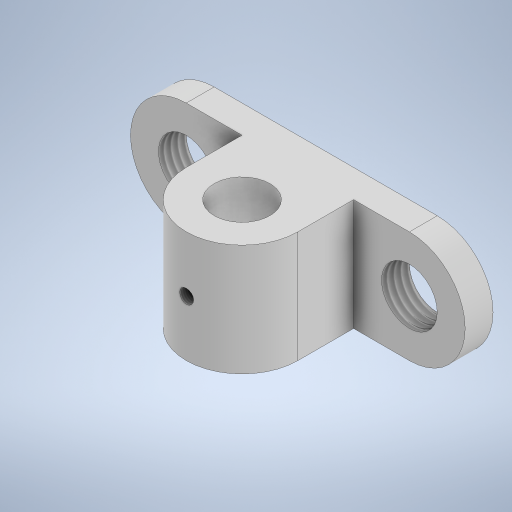
# Autodesk Inventor part: 06022024_ejercicio
Saved by Autodesk Inventor 2024 (Build 280153000, 153)
## iProperties
Created: 2024-02-06
Part Number: 06022024_ejercicio
Material: Generic
Document SubType Name: Modeling
Designer: augus
Density: 1 g/cm^3
Appearance: Default
Author: augus
Autodesk Inventor part; units mm, degrees
ref_plane "YZ Plane" through (0, 0, 0) normal (1, 0, 0) x (0, 1, 0)
ref_plane "XZ Plane" through (0, 0, 0) normal (0, 1, 0) x (-1, 0, 0)
sketch "Sketch2" plane through (0, 0, 0) normal (0, 0, 1) x (1, 0, 0)
  line L0 (-20, 20) -> (20, 20)
  line L1 (20, 20) -> (20, -20)
  line L2 (20, -20) -> (-20, -20)
  line L3 (-20, -20) -> (-20, 20)
  line L4 (-20, 20) -> (20, -20) construction
  line L5 (20, 20) -> (-20, -20) construction
  point P0 (0, 0)
  dimension "d5" = 40
  dimension "d6" = 40
  constraints: 12 end point, 2 midpoint, 2 parallel, 1 horizontal, 1 perpendicular
  measures "d5" distance of L1.end L2.end
  measures "d6" distance of L0.end L1.end
extrude "Extrusion2" add sketch "Sketch2" along normal blind 50
sketch "Sketch3" plane through (20, -20, 0) normal (1, 0, 0) x (0, 0, -1)
  line L0 (0, 40) -> (-50, 40) projected
  line L1 (0, 0) -> (-50, 0) projected
  line L2 (0, 40) -> (-10, 40)
  line L3 (-10, 40) -> (-10, 0)
  line L4 (-10, 0) -> (0, 0)
  line L5 (0, 0) -> (0, 40)
  point P0 (0, 20)
  dimension "d9" = 10
  constraints: 8 end point, 2 parallel, 1 horizontal, 1 perpendicular, 1 point on line
  measures "d9" distance of L4.end L3.end
extrude "Extrusion3" add sketch "Sketch3" along normal blind 40
sketch "Sketch4" plane through (-20, -20, 0) normal (-1, 0, 0) x (0, 0, 1)
  line L0 (0, 40) -> (0, 0) projected
  line L1 (0, 40) -> (50, 40) projected
  line L2 (0, 0) -> (10, 0)
  line L3 (10, 0) -> (10, 40)
  line L4 (10, 40) -> (0, 40)
  line L5 (0, 40) -> (0, 0)
  point P0 (0, 20)
  dimension "d13" = 10
  constraints: 8 end point, 2 parallel, 1 horizontal, 1 perpendicular, 1 point on line
  measures "d13" distance of L4.end L3.end
extrude "Extrusion4" add sketch "Sketch4" along normal blind 40
sketch "Sketch5" plane through (-20, -20, 10) normal (0, 0, 1) x (1, 0, 0)
  line L0 (0, 40) -> (0, 0) projected
  line L1 (-40, 0) -> (80, 0) projected
  line L2 (-20, 40) -> (-40, 40)
  line L3 (-40, 40) -> (-40, 0)
  line L4 (-40, 0) -> (-20, 0)
  line L5 (0, 0) -> (0, 40)
  circle A0 centre (-20, 20) radius 10
  arc A1 (-20, 40) -> (-20, 0) centre (-20, 20) ccw
  line L6 (0, 40) -> (-40, 40) projected
  line L7 (0, 0) -> (-40, 0) projected
  line L8 (-40, 0) -> (-40, 40) projected
  line L9 (60, 0) -> (80, 0)
  line L10 (80, 0) -> (80, 40)
  line L11 (80, 40) -> (60, 40)
  circle A2 centre (60, 20) radius 10
  arc A3 (60, 0) -> (60, 40) centre (60, 20) ccw
  line L12 (40, 40) -> (80, 40) projected
  line L13 (80, 40) -> (80, 0) projected
  line L14 (40, 0) -> (80, 0) projected
  point P0 (20, 20)
  point P1 (80, 20)
  point P2 (-40, 20)
  constraints: 14 end point, 6 tangent, 5 perpendicular, 4 centre point, 4 point on circle, 3 parallel, 2 coincident, 1 horizontal
extrude "Extrusion5" cut sketch "Sketch5" against normal through all contours A3 L11 L10 | A3 L10 L1 | A1 L3 L2 | L1 L3 A1 | A0 | A2
sketch "Sketch6" plane through (-20, -20, 50) normal (0, -1, 0) x (1, 0, 0)
  line L0 (0, -40) -> (-20, -40) projected
  line L1 (40, -40) -> (40, 0) projected
  line L2 (40, -20) -> (40, 0)
  line L3 (40, 0) -> (0, 0)
  line L4 (0, 0) -> (0, -20)
  arc A0 (40, -20) -> (0, -20) centre (20, -20) ccw
  circle A1 centre (20, -20) radius 10
  line L5 (0, 0) -> (40, 0) projected
  line L6 (40, -40) -> (40, 0) projected
  line L7 (0, -40) -> (0, 0) projected
  point P0 (20, -50)
  point P1 (20, 0)
  dimension "d20" = 20
  constraints: 6 end point, 3 tangent, 2 centre point, 2 point on circle, 1 coincident, 1 parallel, 1 perpendicular
  measures "d20" diameter of A1
extrude "Extrusion6" cut sketch "Sketch6" against normal through all
ref_plane "Work Plane1" through (0, -20, 50) normal (0, 0, -1) x (-1, 0, 0)
sketch "Sketch8" plane through (0, -20, 50) normal (0, 0, -1) x (-1, 0, 0)
  circle A0 centre (0, 20) radius 2.5
  dimension "d31" = 5
  constraints: 1 centre point, 1 coincident
  measures "d31" diameter of A0
extrude "Extrusion7" cut sketch "Sketch8" along normal blind 12
thread "Thread1" size "M20x2.5" class "6H" standard "ANSI Metric M Profile" full length
thread "Thread2" size "M5x0.8" class "6H" standard "ANSI Metric M Profile" full length
thread "Thread3" size "M20x2.5" class "6H" standard "ANSI Metric M Profile" full length
body "Solid2"
